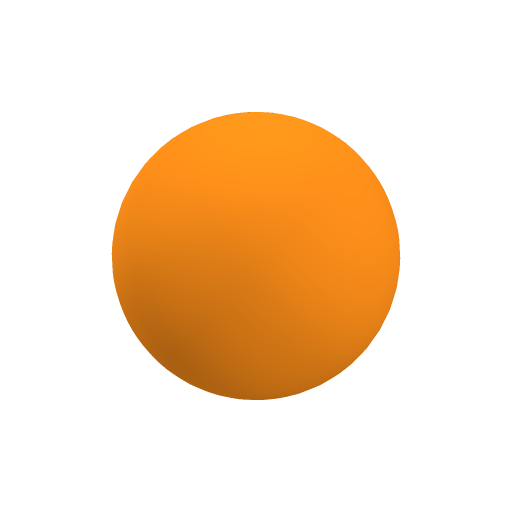
# Autodesk Inventor part: ball_17mm
Saved by Autodesk Inventor 2023 (Build 270158000, 158)
## iProperties
Created: 2024-02-05
Part Number: ball_17mm
Material: PC/ABS Plastic
Document SubType Name: Modeling
Designer: qg3473
Density: 0.357273 g/cm^3
Appearance: Orange
Author: qg3473
Autodesk Inventor part; units mm, degrees
ref_plane "YZ Plane" through (0, 0, 0) normal (1, 0, 0) x (0, 1, 0)
ref_plane "XZ Plane" through (0, 0, 0) normal (0, 1, 0) x (-1, 0, 0)
ref_plane "XY Plane" through (0, 0, 0) normal (0, 0, 1) x (1, 0, 0)
sketch "Sketch1" plane through (0, 0, 0) normal (0, 1, 0) x (-1, 0, 0)
  arc A0 (-8.8832, -18.5241) -> (-8.8832, -1.5241) centre (-8.8832, -10.0241) ccw
  line L0 (-8.8832, -1.5241) -> (-8.8832, -18.5241)
  point P0 (0, 0)
  dimension "d0" = 17
  dimension "d0" = 17
  constraints: 2 end point, 2 point on circle, 1 centre point, 1 vertical
  measures "d0" diameter of A0
revolve "Revolution1" add sketch "Sketch1" angle 360 about axis through (8.8832, 0, -1.5241) along (0, 0, -1)
body "Solid1"
